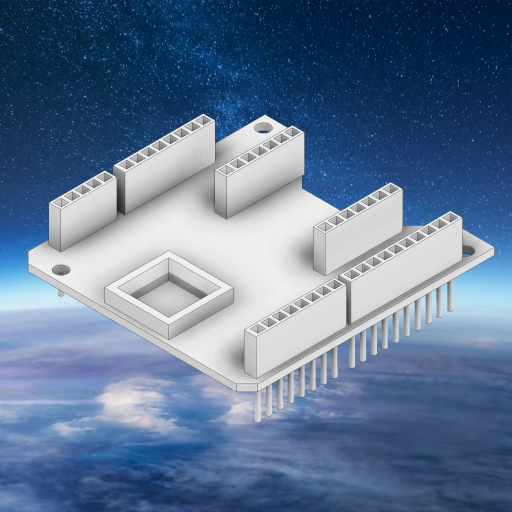
# Autodesk Inventor part: Mti-7 development board
Saved by Autodesk Inventor 2023 (Build 270158000, 158)
## iProperties
Created: 2023-03-23
Part Number: Mti-7 development board
Material: ABS Plastic
Document SubType Name: Modeling
Designer: 310611102
Density: 1.06 g/cm^3
Appearance: Smooth - White
Mass: 7.06573 g
Surface Area: 124.353 cm^2
Volume: 6.66578 cm^3
Author: 310611102
Autodesk Inventor part; units mm, degrees
ref_plane "YZ Plane" through (0, 0, 0) normal (1, 0, 0) x (0, 1, 0)
ref_plane "XZ Plane" through (0, 0, 0) normal (0, 1, 0) x (-1, 0, 0)
ref_plane "XY Plane" through (0, 0, 0) normal (0, 0, 1) x (1, 0, 0)
sketch "Sketch2" plane through (0, 0, 0) normal (0, 1, 0) x (-1, 0, 0)
  line L0 (-26.67, 18.8256) -> (-24.13, 21.3656)
  line L1 (-24.13, 21.3656) -> (24.13, 21.3656)
  line L2 (24.13, 21.3656) -> (26.67, 18.8256)
  line L3 (26.67, 18.8256) -> (26.67, -36.1544)
  line L4 (26.67, -36.1544) -> (18.0269, -36.1544)
  line L5 (18.0269, -36.1544) -> (7.5, -25.6275)
  line L6 (7.5, -25.6275) -> (-7.5, -25.6275)
  line L7 (-7.5, -25.6275) -> (-18.0269, -36.1544)
  line L8 (-18.0269, -36.1544) -> (-26.67, -36.1544)
  line L9 (-26.67, -36.1544) -> (-26.67, 18.8256)
  line L10 (0, -76.2357) -> (0, 55.9303)
  line L11 (0, -102.6689) -> (0, 82.3635) projected
  point P0 (0, 0)
  dimension "d4" = 53.34
  dimension "d5" = 57.52
  dimension "d6" = 2.54
  dimension "d7" = 45
  dimension "d8" = 15
  constraints: 22 end point, 5 perpendicular, 3 point on line, 1 horizontal, 1 horizontal alignment, 1 parallel, 1 symmetric about line, 1 vertical, 3 other
  measures "d4" distance between parallel lines of L9 L3
  measures "d5" distance between parallel lines of L1 L4
  measures "d6" horizontal distance of L1.end L2.end
  measures "d7" angle of L4 L5
  measures "d8" distance of L5.end L6.end
extrude "Extrusion2" add sketch "Sketch2" along normal blind 1.6
sketch "Sketch3" plane through (0, 1.6, 0) normal (0, 1, 0) x (1, 0, 0)
  circle A0 centre (-24.13, 33.2444) radius 1.5
  circle A1 centre (24.13, 31.9744) radius 1.5
  circle A2 centre (-19.05, -18.8256) radius 1.5
  line L0 (-26.67, 36.1544) -> (-26.67, -18.8256) projected
  line L1 (-24.13, -21.3656) -> (24.13, -21.3656) projected
  line L2 (-18.0269, 36.1544) -> (-26.67, 36.1544) projected
  line L3 (26.67, 36.1544) -> (18.0269, 36.1544) projected
  point P0 (0, 0)
  dimension "d11" = 3
  dimension "d12" = 3
  dimension "d13" = 3
  dimension "d14" = 7.62
  dimension "d15" = 2.54
  dimension "d16" = 2.54
  dimension "d17" = 2.91
  dimension "d18" = 4.18
  dimension "d19" = 50.8
  constraints: 3 centre point
  measures "d11" diameter of A0
  measures "d12" diameter of A1
  measures "d13" diameter of A2
  measures "d14" distance from line of L0 A2.centre
  measures "d15" distance from line of L1 A2.centre
  measures "d16" distance from line of L0 A0.centre
  measures "d17" distance from line of A0.centre L2
  measures "d18" distance from line of L3 A1.centre
  measures "d19" distance from line of L0 A1.centre
extrude "Extrusion3" cut sketch "Sketch3" against normal blind 1.6
sketch "Sketch4" plane through (0, 1.6, 0) normal (0, 1, 0) x (1, 0, 0)
  line L0 (-25.53, 20.6744) -> (-22.73, 20.6744)
  line L1 (-22.73, 20.6744) -> (-22.73, -0.3256)
  line L2 (-22.73, -0.3256) -> (-25.53, -0.3256)
  line L3 (-25.53, -0.3256) -> (-25.53, 20.6744)
  line L4 (-25.03, 20.1744) -> (-23.23, 20.1744)
  line L5 (-23.23, 20.1744) -> (-23.23, 18.3744)
  line L6 (-23.23, 18.3744) -> (-25.03, 18.3744)
  line L7 (-25.03, 18.3744) -> (-25.03, 20.1744)
  line L8 (-18.0269, 36.1544) -> (-26.67, 36.1544) projected
  line L9 (-25.03, 15.8344) -> (-25.03, 17.6344)
  line L10 (-25.03, 17.6344) -> (-23.23, 17.6344)
  line L11 (-23.23, 17.6344) -> (-23.23, 15.8344)
  line L12 (-23.23, 15.8344) -> (-25.03, 15.8344)
  line L13 (-25.03, 13.2944) -> (-25.03, 15.0944)
  line L14 (-25.03, 15.0944) -> (-23.23, 15.0944)
  line L15 (-23.23, 15.0944) -> (-23.23, 13.2944)
  line L16 (-23.23, 13.2944) -> (-25.03, 13.2944)
  line L17 (-25.03, 10.7544) -> (-25.03, 12.5544)
  line L18 (-25.03, 12.5544) -> (-23.23, 12.5544)
  line L19 (-23.23, 12.5544) -> (-23.23, 10.7544)
  line L20 (-23.23, 10.7544) -> (-25.03, 10.7544)
  line L21 (-25.03, 8.2144) -> (-25.03, 10.0144)
  line L22 (-25.03, 10.0144) -> (-23.23, 10.0144)
  line L23 (-23.23, 10.0144) -> (-23.23, 8.2144)
  line L24 (-23.23, 8.2144) -> (-25.03, 8.2144)
  line L25 (-25.03, 5.6744) -> (-25.03, 7.4744)
  line L26 (-25.03, 7.4744) -> (-23.23, 7.4744)
  line L27 (-23.23, 7.4744) -> (-23.23, 5.6744)
  line L28 (-23.23, 5.6744) -> (-25.03, 5.6744)
  line L29 (-25.03, 3.1344) -> (-25.03, 4.9344)
  line L30 (-25.03, 4.9344) -> (-23.23, 4.9344)
  line L31 (-23.23, 4.9344) -> (-23.23, 3.1344)
  line L32 (-23.23, 3.1344) -> (-25.03, 3.1344)
  line L33 (-25.03, 0.5944) -> (-25.03, 2.3944)
  line L34 (-25.03, 2.3944) -> (-23.23, 2.3944)
  line L35 (-23.23, 2.3944) -> (-23.23, 0.5944)
  line L36 (-23.23, 0.5944) -> (-25.03, 0.5944)
  line L37 (-25.03, -2.6856) -> (-23.23, -2.6856)
  line L38 (-23.23, -2.6856) -> (-23.23, -4.4856)
  line L39 (-23.23, -4.4856) -> (-25.03, -4.4856)
  line L40 (-25.03, -4.4856) -> (-25.03, -2.6856)
  line L41 (-25.53, -2.1856) -> (-22.73, -2.1856)
  line L42 (-22.73, -2.1856) -> (-22.73, -15.1856)
  line L43 (-22.73, -15.1856) -> (-25.53, -15.1856)
  line L44 (-25.53, -15.1856) -> (-25.53, -2.1856)
  line L45 (-25.03, -7.0256) -> (-25.03, -5.2256)
  line L46 (-25.03, -5.2256) -> (-23.23, -5.2256)
  line L47 (-23.23, -5.2256) -> (-23.23, -7.0256)
  line L48 (-23.23, -7.0256) -> (-25.03, -7.0256)
  line L49 (-25.03, -9.5656) -> (-25.03, -7.7656)
  line L50 (-25.03, -7.7656) -> (-23.23, -7.7656)
  line L51 (-23.23, -7.7656) -> (-23.23, -9.5656)
  line L52 (-23.23, -9.5656) -> (-25.03, -9.5656)
  line L53 (-25.03, -12.1056) -> (-25.03, -10.3056)
  line L54 (-25.03, -10.3056) -> (-23.23, -10.3056)
  line L55 (-23.23, -10.3056) -> (-23.23, -12.1056)
  line L56 (-23.23, -12.1056) -> (-25.03, -12.1056)
  line L57 (-25.03, -14.6456) -> (-25.03, -12.8456)
  line L58 (-25.03, -12.8456) -> (-23.23, -12.8456)
  line L59 (-23.23, -12.8456) -> (-23.23, -14.6456)
  line L60 (-23.23, -14.6456) -> (-25.03, -14.6456)
  line L61 (-26.67, 36.1544) -> (-26.67, -18.8256) projected
  line L62 (-12.83, 28.6644) -> (-10.03, 28.6644)
  line L63 (-10.03, 28.6644) -> (-10.03, 10.6644)
  line L64 (-10.03, 10.6644) -> (-12.83, 10.6644)
  line L65 (-12.83, 10.6644) -> (-12.83, 28.6644)
  line L66 (-12.33, 28.1644) -> (-10.53, 28.1644)
  line L67 (-10.53, 28.1644) -> (-10.53, 26.3644)
  line L68 (-10.53, 26.3644) -> (-12.33, 26.3644)
  line L69 (-12.33, 26.3644) -> (-12.33, 28.1644)
  line L70 (-12.33, 23.8244) -> (-12.33, 25.6244)
  line L71 (-12.33, 25.6244) -> (-10.53, 25.6244)
  line L72 (-10.53, 25.6244) -> (-10.53, 23.8244)
  line L73 (-10.53, 23.8244) -> (-12.33, 23.8244)
  line L74 (-12.33, 21.2844) -> (-12.33, 23.0844)
  line L75 (-12.33, 23.0844) -> (-10.53, 23.0844)
  line L76 (-10.53, 23.0844) -> (-10.53, 21.2844)
  line L77 (-10.53, 21.2844) -> (-12.33, 21.2844)
  line L78 (-12.33, 18.7444) -> (-12.33, 20.5444)
  line L79 (-12.33, 20.5444) -> (-10.53, 20.5444)
  line L80 (-10.53, 20.5444) -> (-10.53, 18.7444)
  line L81 (-10.53, 18.7444) -> (-12.33, 18.7444)
  line L82 (-12.33, 16.2044) -> (-12.33, 18.0044)
  line L83 (-12.33, 18.0044) -> (-10.53, 18.0044)
  line L84 (-10.53, 18.0044) -> (-10.53, 16.2044)
  line L85 (-10.53, 16.2044) -> (-12.33, 16.2044)
  line L86 (-12.33, 13.6644) -> (-12.33, 15.4644)
  line L87 (-12.33, 15.4644) -> (-10.53, 15.4644)
  line L88 (-10.53, 15.4644) -> (-10.53, 13.6644)
  line L89 (-10.53, 13.6644) -> (-12.33, 13.6644)
  line L90 (-12.33, 11.1244) -> (-12.33, 12.9244)
  line L91 (-12.33, 12.9244) -> (-10.53, 12.9244)
  line L92 (-10.53, 12.9244) -> (-10.53, 11.1244)
  line L93 (-10.53, 11.1244) -> (-12.33, 11.1244)
  line L94 (10.53, 26.3644) -> (10.53, 28.1644)
  line L95 (10.53, 28.1644) -> (12.33, 28.1644)
  line L96 (12.33, 28.1644) -> (12.33, 26.3644)
  line L97 (12.33, 26.3644) -> (10.53, 26.3644)
  line L98 (12.33, 23.8244) -> (10.53, 23.8244)
  line L99 (12.33, 25.6244) -> (12.33, 23.8244)
  line L100 (10.53, 23.8244) -> (10.53, 25.6244)
  line L101 (10.53, 25.6244) -> (12.33, 25.6244)
  line L102 (10.03, 28.6644) -> (12.83, 28.6644)
  line L103 (10.53, 23.0844) -> (12.33, 23.0844)
  line L104 (12.33, 21.2844) -> (10.53, 21.2844)
  line L105 (12.33, 23.0844) -> (12.33, 21.2844)
  line L106 (10.53, 21.2844) -> (10.53, 23.0844)
  line L107 (10.53, 20.5444) -> (12.33, 20.5444)
  line L108 (10.03, 10.6644) -> (10.03, 28.6644)
  line L109 (12.83, 28.6644) -> (12.83, 10.6644)
  line L110 (12.33, 20.5444) -> (12.33, 18.7444)
  line L111 (10.53, 18.7444) -> (10.53, 20.5444)
  line L112 (12.33, 18.7444) -> (10.53, 18.7444)
  line L113 (10.53, 18.0044) -> (12.33, 18.0044)
  line L114 (10.53, 16.2044) -> (10.53, 18.0044)
  line L115 (12.33, 18.0044) -> (12.33, 16.2044)
  line L116 (12.33, 16.2044) -> (10.53, 16.2044)
  line L117 (10.53, 15.4644) -> (12.33, 15.4644)
  line L118 (12.83, 10.6644) -> (10.03, 10.6644)
  line L119 (12.33, 11.1244) -> (10.53, 11.1244)
  line L120 (10.53, 11.1244) -> (10.53, 12.9244)
  line L121 (12.33, 12.9244) -> (12.33, 11.1244)
  line L122 (12.33, 13.6644) -> (10.53, 13.6644)
  line L123 (10.53, 13.6644) -> (10.53, 15.4644)
  line L124 (12.33, 15.4644) -> (12.33, 13.6644)
  line L125 (10.53, 12.9244) -> (12.33, 12.9244)
  line L126 (23.23, 27.5184) -> (23.23, 29.3184)
  line L127 (23.23, 29.3184) -> (25.03, 29.3184)
  line L128 (25.03, 29.3184) -> (25.03, 27.5184)
  line L129 (25.03, 27.5184) -> (23.23, 27.5184)
  line L130 (22.73, 29.8184) -> (25.53, 29.8184)
  line L131 (22.73, 3.8184) -> (22.73, 29.8184)
  line L132 (25.53, 29.8184) -> (25.53, 3.8184)
  line L133 (25.53, 3.8184) -> (22.73, 3.8184)
  line L134 (23.23, 24.9784) -> (23.23, 26.7784)
  line L135 (23.23, 26.7784) -> (25.03, 26.7784)
  line L136 (25.03, 26.7784) -> (25.03, 24.9784)
  line L137 (25.03, 24.9784) -> (23.23, 24.9784)
  line L138 (23.23, 22.4384) -> (23.23, 24.2384)
  line L139 (23.23, 24.2384) -> (25.03, 24.2384)
  line L140 (25.03, 24.2384) -> (25.03, 22.4384)
  line L141 (25.03, 22.4384) -> (23.23, 22.4384)
  line L142 (23.23, 19.8984) -> (23.23, 21.6984)
  line L143 (23.23, 21.6984) -> (25.03, 21.6984)
  line L144 (25.03, 21.6984) -> (25.03, 19.8984)
  line L145 (25.03, 19.8984) -> (23.23, 19.8984)
  line L146 (23.23, 17.3584) -> (23.23, 19.1584)
  line L147 (23.23, 19.1584) -> (25.03, 19.1584)
  line L148 (25.03, 19.1584) -> (25.03, 17.3584)
  line L149 (25.03, 17.3584) -> (23.23, 17.3584)
  line L150 (23.23, 14.8184) -> (23.23, 16.6184)
  line L151 (23.23, 16.6184) -> (25.03, 16.6184)
  line L152 (25.03, 16.6184) -> (25.03, 14.8184)
  line L153 (25.03, 14.8184) -> (23.23, 14.8184)
  line L154 (23.23, 12.2784) -> (23.23, 14.0784)
  line L155 (23.23, 14.0784) -> (25.03, 14.0784)
  line L156 (25.03, 14.0784) -> (25.03, 12.2784)
  line L157 (25.03, 12.2784) -> (23.23, 12.2784)
  line L158 (23.23, 9.7384) -> (23.23, 11.5384)
  line L159 (23.23, 11.5384) -> (25.03, 11.5384)
  line L160 (25.03, 11.5384) -> (25.03, 9.7384)
  line L161 (25.03, 9.7384) -> (23.23, 9.7384)
  line L162 (23.23, 7.1984) -> (23.23, 8.9984)
  line L163 (23.23, 8.9984) -> (25.03, 8.9984)
  line L164 (25.03, 8.9984) -> (25.03, 7.1984)
  line L165 (25.03, 7.1984) -> (23.23, 7.1984)
  line L166 (23.23, 4.6584) -> (23.23, 6.4584)
  line L167 (23.23, 6.4584) -> (25.03, 6.4584)
  line L168 (25.03, 6.4584) -> (25.03, 4.6584)
  line L169 (25.03, 4.6584) -> (23.23, 4.6584)
  line L170 (-24.13, -21.3656) -> (24.13, -21.3656) projected
  line L171 (26.67, -18.8256) -> (26.67, 36.1544) projected
  line L172 (22.73, 2.8944) -> (25.53, 2.8944)
  line L173 (25.53, 2.8944) -> (25.53, -18.1056)
  line L174 (25.53, -18.1056) -> (22.73, -18.1056)
  line L175 (22.73, -18.1056) -> (22.73, 2.8944)
  line L176 (23.23, 2.3944) -> (25.03, 2.3944)
  line L177 (25.03, 2.3944) -> (25.03, 0.5944)
  line L178 (25.03, 0.5944) -> (23.23, 0.5944)
  line L179 (23.23, 0.5944) -> (23.23, 2.3944)
  line L180 (23.23, -1.9456) -> (23.23, -0.1456)
  line L181 (23.23, -0.1456) -> (25.03, -0.1456)
  line L182 (25.03, -0.1456) -> (25.03, -1.9456)
  line L183 (25.03, -1.9456) -> (23.23, -1.9456)
  line L184 (23.23, -4.4856) -> (23.23, -2.6856)
  line L185 (23.23, -2.6856) -> (25.03, -2.6856)
  line L186 (25.03, -2.6856) -> (25.03, -4.4856)
  line L187 (25.03, -4.4856) -> (23.23, -4.4856)
  line L188 (23.23, -7.0256) -> (23.23, -5.2256)
  line L189 (23.23, -5.2256) -> (25.03, -5.2256)
  line L190 (25.03, -5.2256) -> (25.03, -7.0256)
  line L191 (25.03, -7.0256) -> (23.23, -7.0256)
  line L192 (23.23, -9.5656) -> (23.23, -7.7656)
  line L193 (23.23, -7.7656) -> (25.03, -7.7656)
  line L194 (25.03, -7.7656) -> (25.03, -9.5656)
  line L195 (25.03, -9.5656) -> (23.23, -9.5656)
  line L196 (23.23, -12.1056) -> (23.23, -10.3056)
  line L197 (23.23, -10.3056) -> (25.03, -10.3056)
  line L198 (25.03, -10.3056) -> (25.03, -12.1056)
  line L199 (25.03, -12.1056) -> (23.23, -12.1056)
  line L200 (23.23, -14.6456) -> (23.23, -12.8456)
  line L201 (23.23, -12.8456) -> (25.03, -12.8456)
  line L202 (25.03, -12.8456) -> (25.03, -14.6456)
  line L203 (25.03, -14.6456) -> (23.23, -14.6456)
  line L204 (23.23, -17.1856) -> (23.23, -15.3856)
  line L205 (23.23, -15.3856) -> (25.03, -15.3856)
  line L206 (25.03, -15.3856) -> (25.03, -17.1856)
  line L207 (25.03, -17.1856) -> (23.23, -17.1856)
  line L208 (7.5, 25.6275) -> (-7.5, 25.6275) projected
  circle A0 centre (-24.13, 33.2444) radius 1.5 projected
  point P0 (0, 0)
  point P1 (-25.03, 19.2744)
  point P2 (-25.03, 16.7344)
  point P3 (-25.03, 14.1944)
  point P4 (-25.03, 11.6544)
  point P5 (-25.03, 9.1144)
  point P6 (-25.03, 6.5744)
  point P7 (-25.03, 4.0344)
  point P8 (-25.03, 1.4944)
  point P9 (-25.03, -3.5856)
  point P10 (-25.03, -6.1256)
  point P11 (-25.03, -8.6656)
  point P12 (-25.03, -11.2056)
  point P13 (-25.03, -13.7456)
  point P14 (-24.13, -14.6456)
  point P15 (-11.43, 26.3644)
  point P16 (-12.33, 27.2644)
  point P17 (-12.33, 24.7244)
  point P18 (-11.43, 23.8244)
  point P19 (-12.33, 22.1844)
  point P20 (-11.43, 21.2844)
  point P21 (-12.33, 19.6444)
  point P22 (-11.43, 18.7444)
  point P23 (-12.33, 17.1044)
  point P24 (-11.43, 16.2044)
  point P25 (-12.33, 14.5644)
  point P26 (-11.43, 13.6644)
  point P27 (-12.33, 12.0244)
  point P28 (-11.43, 11.1244)
  point P29 (10.53, 27.2644)
  point P30 (11.43, 26.3644)
  point P31 (11.43, 23.8244)
  point P32 (10.53, 24.7244)
  point P33 (10.53, 22.1844)
  point P34 (11.43, 21.2844)
  point P35 (10.53, 19.6444)
  point P36 (11.43, 18.7444)
  point P37 (10.53, 17.1044)
  point P38 (11.43, 16.2044)
  point P39 (11.43, 11.1244)
  point P40 (10.53, 12.0244)
  point P41 (11.43, 13.6644)
  point P42 (10.53, 14.5644)
  point P43 (25.03, 5.5584)
  point P44 (24.13, 4.6584)
  point P45 (23.23, -16.2856)
  point P46 (24.13, -17.1856)
  point P47 (0, 25.6275)
  dimension "d22" = 1.8
  dimension "d23" = 1.8
  dimension "d24" = 2.8
  dimension "d25" = 0.5
  dimension "d26" = 0.5
  dimension "d27" = 16.88
  dimension "d30" = 2.54
  dimension "d35" = 21
  dimension "d40" = 1.8
  dimension "d41" = 1.8
  dimension "d42" = 2.8
  dimension "d43" = 0.5
  dimension "d44" = 0.5
  dimension "d45" = 39.74
  dimension "d48" = 2.54
  dimension "d53" = 2.54
  dimension "d54" = 13
  dimension "d63" = 1.8
  dimension "d64" = 1.8
  dimension "d65" = 2.8
  dimension "d66" = 0.5
  dimension "d68" = 18
  dimension "d83" = 0.5
  dimension "d84" = 15.24
  dimension "d85" = 8.89
  dimension "d88" = 2.54
  dimension "d95" = 22.86
  dimension "d116" = 0.5
  dimension "d117" = 0.5
  dimension "d118" = 2.8
  dimension "d119" = 26
  dimension "d120" = 1.8
  dimension "d121" = 1.8
  dimension "d124" = 2.54
  dimension "d129" = 26.924
  dimension "d130" = 2.54
  dimension "d158" = 2.8
  dimension "d159" = 1.8
  dimension "d160" = 1.8
  dimension "d161" = 0.5
  dimension "d162" = 0.5
  dimension "d165" = 2.54
  dimension "d172" = 2.54
  dimension "d177" = 5.08
  dimension "d178" = 21
  dimension "d179" = 2.54
  dimension "d276" = 24.13
  constraints: 408 end point, 16 parallel, 10 midpoint, 9 horizontal, 8 perpendicular, 8 vertical, 5 collinear, 361 other
  measures "d22" distance of L4.start L4.end
  measures "d23" distance of L4.end L5.end
  measures "d24" distance of L0.start L0.end
  measures "d25" distance from line of point (-25.03, 19.274) L3
  measures "d26" distance between parallel lines of L4 L0
  measures "d27" distance from line of L8 point (-25.03, 19.274)
  measures "d30" distance of L6.end L9.start
  measures "d35" distance of L2.end L0.start
  measures "d40" distance of L37.start L37.end
  measures "d41" distance of L37.end L38.end
  measures "d42" distance of L41.start L41.end
  measures "d43" distance between parallel lines of L44 L40
  measures "d44" distance between parallel lines of L41 L37
  measures "d45" distance from line of L8 point (-25.03, -3.586)
  measures "d48" distance of L39.end L45.start
  measures "d53" distance from line of L61 point (-24.13, -14.646)
  measures "d54" distance of L43.end L41.start
  measures "d63" distance of L69.end L66.end
  measures "d64" distance of L66.end L67.end
  measures "d65" distance of L65.end L62.end
  measures "d66" distance between parallel lines of L66 L62
  measures "d68" distance of L65.start L65.end
  measures "d83" distance between parallel lines of L69 L65
  measures "d84" distance from line of L61 point (-11.43, 26.364)
  measures "d85" distance from line of L8 point (-12.33, 27.264)
  measures "d88" distance of L69.start L70.start
  measures "d95" distance of L69.start L94.start
  measures "d116" distance between parallel lines of L131 L126
  measures "d117" distance between parallel lines of L127 L130
  measures "d118" distance between parallel lines of L132 L131
  measures "d119" distance between parallel lines of L133 L130
  measures "d120" distance of L126.start L126.end
  measures "d121" distance of L126.end L127.end
  measures "d124" distance of L126.start L134.start
  measures "d129" distance from line of L170 point (25.03, 5.558)
  measures "d130" distance from line of L171 point (24.13, 4.658)
  measures "d158" distance of L172.start L172.end
  measures "d159" distance of L176.start L176.end
  measures "d160" distance of L178.end L176.start
  measures "d161" distance between parallel lines of L175 L179
  measures "d162" distance between parallel lines of L172 L176
  measures "d165" distance of L178.end L180.start
  measures "d172" distance of L200.start L204.start
  measures "d177" distance from line of L170 point (23.23, -16.286)
  measures "d178" distance of L174.end L172.start
  measures "d179" distance from line of L171 point (24.13, -17.186)
  measures "d276" horizontal distance of point (0, 25.627) A0.centre
extrude "Extrusion4" add sketch "Sketch4" along normal blind 8.51 contours L0 L1 L2 L3 | L41 L42 L43 L44 | L62 L63 L64 L65 | L102 L109 L118 L108 | L130 L132 L133 L131 | L172 L173 L174 L175
sketch "Sketch5" plane through (0, 1.6, 0) normal (0, 1, 0) x (1, 0, 0)
  circle A0 centre (-24.13, -13.7456) radius 0.5
  line L0 (-23.23, -12.8456) -> (-23.23, -14.6456) projected
  line L1 (-25.03, -12.8456) -> (-23.23, -12.8456) projected
  line L2 (-24.13, -13.7456) -> (-24.13, -11.6479)
  circle A1 centre (-24.13, -11.2056) radius 0.5
  circle A2 centre (-24.13, -8.6656) radius 0.5
  circle A3 centre (-24.13, -6.1256) radius 0.5
  circle A4 centre (-24.13, -3.5856) radius 0.5
  circle A5 centre (-24.13, 1.4944) radius 0.5
  line L3 (-25.03, 2.3944) -> (-23.23, 2.3944) projected
  line L4 (-23.23, 2.3944) -> (-23.23, 0.5944) projected
  circle A6 centre (-24.13, 4.0344) radius 0.5
  circle A7 centre (-24.13, 6.5744) radius 0.5
  circle A8 centre (-24.13, 9.1144) radius 0.5
  circle A9 centre (-24.13, 11.6544) radius 0.5
  circle A10 centre (-24.13, 14.1944) radius 0.5
  circle A11 centre (-24.13, 16.7344) radius 0.5
  circle A12 centre (-24.13, 19.2744) radius 0.5
  circle A13 centre (-11.43, 12.0244) radius 0.5
  circle A14 centre (11.43, 12.0244) radius 0.5
  circle A15 centre (24.13, 5.5584) radius 0.5
  circle A16 centre (24.13, -16.2856) radius 0.5
  line L5 (-10.53, 12.9244) -> (-10.53, 11.1244) projected
  line L6 (-12.33, 12.9244) -> (-10.53, 12.9244) projected
  line L7 (12.33, 12.9244) -> (12.33, 11.1244) projected
  line L8 (10.53, 12.9244) -> (12.33, 12.9244) projected
  line L9 (23.23, 6.4584) -> (25.03, 6.4584) projected
  line L10 (23.23, 4.6584) -> (23.23, 6.4584) projected
  line L11 (23.23, -17.1856) -> (23.23, -15.3856) projected
  line L12 (23.23, -15.3856) -> (25.03, -15.3856) projected
  circle A17 centre (-11.43, 14.5644) radius 0.5
  circle A18 centre (-11.43, 17.1044) radius 0.5
  circle A19 centre (-11.43, 19.6444) radius 0.5
  circle A20 centre (-11.43, 22.1844) radius 0.5
  circle A21 centre (-11.43, 24.7244) radius 0.5
  circle A22 centre (-11.43, 27.2644) radius 0.5
  circle A23 centre (11.43, 14.5644) radius 0.5
  circle A24 centre (11.43, 17.1044) radius 0.5
  circle A25 centre (11.43, 19.6444) radius 0.5
  circle A26 centre (11.43, 22.1844) radius 0.5
  circle A27 centre (11.43, 24.7244) radius 0.5
  circle A28 centre (11.43, 27.2644) radius 0.5
  circle A29 centre (24.13, 8.0984) radius 0.5
  circle A30 centre (24.13, 10.6384) radius 0.5
  circle A31 centre (24.13, 13.1784) radius 0.5
  circle A32 centre (24.13, 15.7184) radius 0.5
  circle A33 centre (24.13, 18.2584) radius 0.5
  circle A34 centre (24.13, 20.7984) radius 0.5
  circle A35 centre (24.13, 23.3384) radius 0.5
  circle A36 centre (24.13, 25.8784) radius 0.5
  circle A37 centre (24.13, 28.4184) radius 0.5
  circle A38 centre (24.13, -13.7456) radius 0.5
  circle A39 centre (24.13, -11.2056) radius 0.5
  circle A40 centre (24.13, -8.6656) radius 0.5
  circle A41 centre (24.13, -6.1256) radius 0.5
  circle A42 centre (24.13, -3.5856) radius 0.5
  circle A43 centre (24.13, -1.0456) radius 0.5
  circle A44 centre (24.13, 1.4944) radius 0.5
  point P0 (0, 0)
  point P1 (-23.23, -13.7456)
  point P2 (-24.13, -12.8456)
  point P3 (-24.13, 2.3944)
  point P4 (-23.23, 1.4944)
  point P5 (-10.53, 12.0244)
  point P6 (-11.43, 12.9244)
  point P7 (12.33, 12.0244)
  point P8 (11.43, 12.9244)
  point P9 (24.13, 6.4584)
  point P10 (23.23, 5.5584)
  point P11 (23.23, -16.2856)
  point P12 (24.13, -15.3856)
  dimension "d182" = 1
  dimension "d185" = 2.54
  dimension "d194" = 1
  dimension "d197" = 2.54
  dimension "d236" = 2.54
  dimension "d241" = 1
  dimension "d242" = 1
  dimension "d243" = 1
  dimension "d244" = 1
  dimension "d247" = 2.54
  dimension "d254" = 2.54
  dimension "d261" = 2.54
  constraints: 45 centre point, 12 midpoint, 7 vertical, 6 horizontal alignment, 6 vertical alignment, 2 end point, 78 other
  measures "d182" diameter of A0
  measures "d185" distance of L2.start A1.centre
  measures "d194" diameter of A5
  measures "d197" distance of A5.centre A6.centre
  measures "d236" distance of A13.centre A17.centre
  measures "d241" diameter of A13
  measures "d242" diameter of A14
  measures "d243" diameter of A15
  measures "d244" diameter of A16
  measures "d247" distance of A14.centre A23.centre
  measures "d254" distance of A15.centre A29.centre
  measures "d261" distance of A16.centre A38.centre
extrude "Extrusion5" add sketch "Sketch5" against normal blind 10
sketch "Sketch6" plane through (0, 1.6, 0) normal (0, 1, 0) x (1, 0, 0)
  line L0 (-7.5, -5.3345) -> (7.5, -5.3345)
  line L1 (7.5, -5.3345) -> (7.5, -20.3345)
  line L2 (7.5, -20.3345) -> (-7.5, -20.3345)
  line L3 (-7.5, -20.3345) -> (-7.5, -5.3345)
  line L4 (-7.5, -5.3345) -> (7.5, -20.3345) construction
  line L5 (7.5, -5.3345) -> (-7.5, -20.3345) construction
  line L6 (-4.5, -8.3345) -> (4.5, -8.3345)
  line L7 (4.5, -8.3345) -> (4.5, -17.3345)
  line L8 (4.5, -17.3345) -> (-4.5, -17.3345)
  line L9 (-4.5, -17.3345) -> (-4.5, -8.3345)
  line L10 (-4.5, -8.3345) -> (4.5, -17.3345) construction
  line L11 (4.5, -8.3345) -> (-4.5, -17.3345) construction
  point P0 (0, 0)
  point P1 (0, -12.8345)
  dimension "d268" = 15
  dimension "d269" = 15
  dimension "d270" = 3
  constraints: 24 end point, 4 midpoint, 4 parallel, 2 horizontal, 2 perpendicular, 1 point on line
  measures "d268" distance of L0.end L1.end
  measures "d269" distance of L0.start L0.end
  measures "d270" distance between parallel lines of L1 L7
extrude "Extrusion6" add sketch "Sketch6" along normal blind 3
chamfer "Chamfer1" distance 1.5 angle 45 4 edges at (-4.5, 4.6, 12.8345) (0, 4.6, 8.3345) (4.5, 4.6, 12.8345) (0, 4.6, 17.3345)
body "Solid2"
